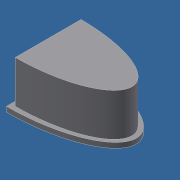
# Autodesk Inventor part: P1704_019_button_triangle_cap
Saved by Autodesk Inventor 2019 (Build 230136000, 136)
## iProperties
Created: 2019-06-03
Part Number: P1704_019_button_triangle_cap
Project: Nom Projet
Material: .
Description: Nom pièce
Document SubType Name: Modeling
Designer: Adel.KAHRIMANOVIC
Authority: brut Ø
Density: 0.001 g/cm^3
Appearance: Par défaut
Author: Adel.KAHRIMANOVIC
Material number: ---
Autodesk Inventor part; units mm, degrees
ref_plane "Plan YZ" through (0, 0, 0) normal (1, 0, 0) x (0, 1, 0)
ref_plane "Plan XZ" through (0, 0, 0) normal (0, 1, 0) x (-1, 0, 0)
ref_plane "Plan XY" through (0, 0, 0) normal (0, 0, 1) x (1, 0, 0)
sketch "Esquisse1" plane through (0, 0, 0) normal (0, 0, 1) x (1, 0, 0)
  line L0 (0, 11.8) -> (0, 0)
  ellipse E0 centre (0, 5.9) end of major axis (14.65, 5.9) minor radius 5.9
  dimension "d13" = 14.65
  dimension "d1" = 11.8
  constraints: 2 end point, 1 midpoint, 1 vertical, 4 other
  measures "d1" distance of L0.start L0.end
extrude "Extrusion3" add sketch "Esquisse1" along normal blind 0.8 contours E0 L0 picked at (3.5971, 4.141)
sketch "Esquisse7" plane through (0, 0, 0.8) normal (0, 0, 1) x (1, 0, 0)
  ellipse E0 centre (0.7, 5.9) end of major axis (13.95, 5.9) minor radius 5.2
  line L0 (0.7, 11.1) -> (0.7, 0.7)
  line L1 (0, 11.8) -> (0, 0) projected
  line L2 (0.7, 11.7933) -> (0.7, 11.1) construction
  line L3 (0.7, 0.7) -> (0.7, 0.0067) construction
  ellipse E1 centre (0, 5.9) end of major axis (14.65, 5.9) minor radius 5.9 (0, 0) -> (0, 11.8) ccw projected
  dimension "d16" = 13.25
  dimension "d17" = 10.4
  dimension "d18" = 0.7
  constraints: 6 end point, 2 collinear, 2 vertical, 1 midpoint, 7 other
  measures "d17" distance of L0.start L0.end
  measures "d18" distance between parallel lines of L1 L0
extrude "Extrusion4" add sketch "Esquisse7" along normal blind 6.7 contours E0 L0
sketch "Esquisse8" plane through (0, 0, 0) normal (0, 0, -1) x (-1, 0, 0)
  circle A0 centre (-5.3, 5.9) radius 4.3
  line L0 (0, 11.8) -> (0, 0) projected
  line L1 (2.2688, 5.9) -> (-1.7595, 5.9) construction
  line L2 (0, 0) -> (0, 5.9) construction
  line L3 (0, 5.9) -> (0, 11.8) construction
  dimension "d21" = 8.6
  dimension "d22" = 5.3
  constraints: 6 end point, 3 point on line, 1 centre point, 1 collinear, 1 horizontal, 1 perpendicular
  measures "d21" diameter of A0
  measures "d22" distance from line of L0 A0.centre
extrude "Extrusion5" cut sketch "Esquisse8" against normal blind 3
